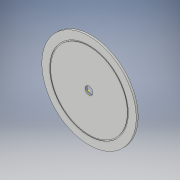
# Autodesk Inventor part: PlateCenter
Saved by Autodesk Inventor 2019 (Build 230136000, 136)
## iProperties
Created: 2019-05-09
Part Number: PlateCenter
Material: Generic
Document SubType Name: Modeling
Designer: samson.bailor
Density: 1 g/cm^3
Appearance: Default
Author: samson.bailor
Autodesk Inventor part; units mm, degrees
ref_plane "YZ Plane" through (0, 0, 0) normal (1, 0, 0) x (0, 1, 0)
ref_plane "XZ Plane" through (0, 0, 0) normal (0, 1, 0) x (-1, 0, 0)
ref_plane "XY Plane" through (0, 0, 0) normal (0, 0, 1) x (1, 0, 0)
sketch "Sketch1" plane through (0, 0, 0) normal (0, 0, 1) x (1, 0, 0)
  circle A0 centre (0, 0) radius 152.4
  circle A1 centre (0, 0) radius 12.7
  dimension "d0" = 304.8
  dimension "d1" = 25.4
  constraints: 2 centre point, 2 coincident
  measures "d0" diameter of A0
  measures "d1" diameter of A1
extrude "Extrusion1" add sketch "Sketch1" along normal blind 6.35
sketch "Sketch2" plane through (0, 0, 6.35) normal (0, 0, 1) x (1, 0, 0)
  point P0 (0, 0)
sketch "Sketch3" plane through (0, 0, 6.35) normal (0, 0, 1) x (1, 0, 0)
  circle A0 centre (0, 0) radius 127
  circle A1 centre (0, 0) radius 123.825
  dimension "d4" = 254
  dimension "d5" = 247.65
  constraints: 2 centre point, 2 coincident
  measures "d4" diameter of A0
  measures "d5" diameter of A1
extrude "Extrusion2" cut sketch "Sketch3" against normal blind 1.27
sketch "Sketch4" plane through (0, 0, 0) normal (0, 0, -1) x (-1, 0, 0)
  circle A0 centre (0, 0) radius 152.4
  circle A1 centre (0, 0) radius 127
  circle A2 centre (0, 0) radius 123.825
  dimension "d8" = 254
  dimension "d9" = 247.65
  constraints: 3 centre point, 3 coincident
  measures "d8" diameter of A1
  measures "d9" diameter of A2
extrude "Extrusion3" cut sketch "Sketch4" against normal blind 1.27 contours A1
sketch "Sketch5" plane through (0, 0, 6.35) normal (0, 0, 1) x (1, 0, 0)
  circle A0 centre (0, 0) radius 12.7 projected
  line L0 (0, 12.7) -> (0, 13.208)
  line L1 (0, 13.208) -> (1.27, 13.208)
  line L2 (0, 13.208) -> (-1.27, 13.208)
  line L3 (-1.27, 13.208) -> (-1.27, 12.2678)
  line L4 (1.27, 13.208) -> (1.27, 12.2294)
  arc A1 (1.27, 12.6363) -> (-1.27, 12.6363) centre (0, 0) ccw
  dimension "d12" = 0.508
  dimension "d15" = 1.27
  dimension "d16" = 1.27
  constraints: 10 end point, 6 point on circle, 2 horizontal, 2 point on line, 2 vertical, 1 centre point, 1 perpendicular
  measures "d12" distance of L0.start L0.end
  measures "d15" distance of L0.end L1.end
  measures "d16" distance of L0.end L2.end
extrude "Extrusion4" cut sketch "Sketch5" against normal blind 1.27 contours A0 L0 L1 L4 | L3 L2 L0 A0
body "Solid1"
